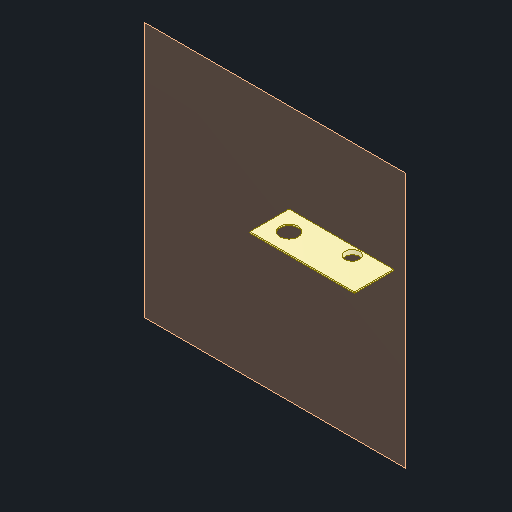
# Autodesk Inventor part: right_hold
Saved by Autodesk Inventor 2023 (Build 270158000, 158)
## iProperties
Created: 2024-05-18
Part Number: right_hold
Material: Nylon 6/6
Document SubType Name: Modeling
Designer: szymo
Density: 1.13 g/cm^3
Appearance: Nylon 6
Mass: 2.76791 g
Surface Area: 49.1971 cm^2
Volume: 2.44948 cm^3
Author: szymo
Autodesk Inventor part; units mm, degrees
ref_plane "YZ Plane" through (0, 0, 0) normal (1, 0, 0) x (0, 1, 0)
ref_plane "XZ Plane" through (0, 0, 0) normal (0, 1, 0) x (-1, 0, 0)
ref_plane "XY Plane" through (0, 0, 0) normal (0, 0, 1) x (1, 0, 0)
ref_plane "Work Plane1" through (0, 0, 0) normal (0, 0, 1) x (1, 0, 0)
sketch "Sketch1" plane through (0, 0, 0) normal (0, 0, 1) x (1, 0, 0)
  line L0 (-71, -74) -> (-71, -89) projected
  line L1 (-71, -89) -> (41, -89) projected
  line L2 (41, -89) -> (41, -30.5) projected
  line L3 (41, -30.5) -> (91, -30.5) projected
  line L4 (91, -30.5) -> (91, 30.5) projected
  line L5 (91, 30.5) -> (41, 30.5) projected
  line L6 (41, 30.5) -> (41, 89) projected
  line L7 (41, 89) -> (-71, 89) projected
  line L8 (-71, 89) -> (-71, 74) projected
  line L9 (-71, 74) -> (-87, 74) projected
  line L10 (-87, 74) -> (-87, 89) projected
  line L11 (-87, 89) -> (-91, 89) projected
  line L12 (-91, 89) -> (-91, -89) projected
  line L13 (-91, -89) -> (-87, -89) projected
  line L14 (-87, -89) -> (-87, -74) projected
  line L15 (-87, -74) -> (-71, -74) projected
  line L16 (91, 29.5) -> (11, 29.5)
  line L17 (11, 29.5) -> (11, 28.5)
  line L18 (11, 28.5) -> (91, 28.5)
  line L19 (91, 28.5) -> (91, 29.5)
  line L20 (71.5, 26) -> (60.5, 26) projected
  line L21 (12, 37) -> (40, 37) projected
  line L22 (11, 8.5) -> (11, 9.5)
  point P0 (0, 0)
  dimension "d0" = 1
  dimension "d1" = 2.5
  dimension "d2" = 1
  dimension "d14" = 0
  constraints: 10 end point, 2 parallel, 1 horizontal, 1 perpendicular, 1 point on line, 1 vertical, 2 other
  measures "d0" distance between parallel lines of L5 L16
  measures "d1" distance between parallel lines of L18 L20
  measures "d2" distance between parallel lines of L16 L18
  measures "d14" distance between parallel lines of L22 L17
ref_plane "Work Plane2" through (11, 8.5, 30) normal (0, 0, 1) x (1, 0, 0)
extrude "Extrusion1" add sketch "Sketch1" along normal up to surface (30 mm away) contours L18 L17 L16 L4
sketch "Sketch2" plane through (11, 28.5, 0) normal (0, -1, 0) x (1, 0, 0)
  circle A0 centre (55, 6.5) radius 5.5 projected
  arc A1 (12.5575, 17.9943) -> (10.6437, 18.8944) centre (9.6132, 14.2185) ccw projected
  arc A2 (10.6437, 18.8944) -> (10.0881, 18.165) centre (15, 15) ccw projected
  arc A3 (10.0881, 18.165) -> (11.4644, 16.5591) centre (14.322, 20.4008) ccw projected
  arc A4 (11.4644, 16.5591) -> (11.264, 15.9868) centre (15, 15) ccw projected
  arc A5 (11.264, 15.9868) -> (9.1866, 15.59) centre (11.1013, 11.2015) ccw projected
  arc A6 (9.1866, 15.59) -> (9.1659, 14.6734) centre (15, 15) ccw projected
  arc A7 (9.1659, 14.6734) -> (11.2232, 14.1831) centre (11.277, 18.9709) ccw projected
  arc A8 (11.2232, 14.1831) -> (11.3975, 13.6024) centre (15, 15) ccw projected
  arc A9 (11.3975, 13.6024) -> (9.95, 12.0603) centre (14.0786, 9.6353) ccw projected
  arc A10 (9.95, 12.0603) -> (10.4721, 11.3065) centre (15, 15) ccw projected
  arc A11 (10.4721, 11.3065) -> (12.4247, 12.1192) centre (9.654, 16.0242) ccw projected
  arc A12 (12.4247, 12.1192) -> (12.907, 11.7518) centre (15, 15) ccw projected
  arc A13 (12.907, 11.7518) -> (12.6424, 9.6535) centre (17.4078, 10.1183) ccw projected
  arc A14 (12.6424, 9.6535) -> (13.5078, 9.3505) centre (15, 15) ccw projected
  arc A15 (13.5078, 9.3505) -> (14.6098, 11.1556) centre (10.073, 12.6863) ccw projected
  arc A16 (14.6098, 11.1556) -> (15.216, 11.1419) centre (15, 15) ccw projected
  arc A17 (15.216, 11.1419) -> (16.2353, 9.2888) centre (19.8174, 12.4659) ccw projected
  arc A18 (16.2353, 9.2888) -> (17.1135, 9.5523) centre (15, 15) ccw projected
  arc A19 (17.1135, 9.5523) -> (16.944, 11.6605) centre (12.3739, 10.2321) ccw projected
  arc A20 (16.944, 11.6605) -> (17.4425, 12.0057) centre (15, 15) ccw projected
  arc A21 (17.4425, 12.0057) -> (19.3563, 11.1056) centre (20.3868, 15.7815) ccw projected
  arc A22 (19.3563, 11.1056) -> (19.9119, 11.835) centre (15, 15) ccw projected
  arc A23 (19.9119, 11.835) -> (18.5356, 13.4409) centre (15.678, 9.5992) ccw projected
  arc A24 (18.5356, 13.4409) -> (18.736, 14.0132) centre (15, 15) ccw projected
  arc A25 (18.736, 14.0132) -> (20.8134, 14.41) centre (18.8987, 18.7985) ccw projected
  arc A26 (20.8134, 14.41) -> (20.8341, 15.3266) centre (15, 15) ccw projected
  arc A27 (20.8341, 15.3266) -> (18.7768, 15.8169) centre (18.723, 11.0291) ccw projected
  arc A28 (18.7768, 15.8169) -> (18.6025, 16.3976) centre (15, 15) ccw projected
  arc A29 (18.6025, 16.3976) -> (20.05, 17.9397) centre (15.9214, 20.3647) ccw projected
  arc A30 (20.05, 17.9397) -> (19.5279, 18.6935) centre (15, 15) ccw projected
  arc A31 (19.5279, 18.6935) -> (17.5753, 17.8808) centre (20.346, 13.9758) ccw projected
  arc A32 (17.5753, 17.8808) -> (17.093, 18.2482) centre (15, 15) ccw projected
  arc A33 (17.093, 18.2482) -> (17.3576, 20.3465) centre (12.5922, 19.8817) ccw projected
  arc A34 (17.3576, 20.3465) -> (16.4922, 20.6495) centre (15, 15) ccw projected
  arc A35 (16.4922, 20.6495) -> (15.3902, 18.8444) centre (19.927, 17.3137) ccw projected
  arc A36 (15.3902, 18.8444) -> (14.784, 18.8581) centre (15, 15) ccw projected
  arc A37 (14.784, 18.8581) -> (13.7647, 20.7112) centre (10.1826, 17.5341) ccw projected
  arc A38 (13.7647, 20.7112) -> (12.8865, 20.4477) centre (15, 15) ccw projected
  arc A39 (12.8865, 20.4477) -> (13.056, 18.3395) centre (17.6261, 19.7679) ccw projected
  arc A40 (13.056, 18.3395) -> (12.5575, 17.9943) centre (15, 15) ccw projected
  circle A41 centre (15, 15) radius 5.8433
  circle A42 centre (15, 15) radius 7
  point P0 (-11, 0)
  dimension "d12" = 11.6865
  dimension "d13" = 14
  constraints: 2 centre point, 2 coincident
  measures "d12" diameter of A41
  measures "d13" diameter of A42
extrude "Extrusion2" cut sketch "Sketch2" against normal up to next contours A0 | A40 A39 A38 A37 A36 A35 A34 A33 A32 A31 A30 A29 A28 A27 A26 A25 A24 A23 A22 A21 A20 A19 A18 A17 A16 A15 A14 A13 A12 A11 A10 A9 A8 A7 A6 A5 A4 A3 A2 A1 | A1 A41 A39 A40 | A3 A4 A5 A41 | A41 A35 A36 A37 | A7 A8 A9 A41 | A41 A31 A32 A33 | A11 A12 A13 A41 | A41 A27 A28 A29 | A15 A16 A17 A41 | A19 A20 A21 A41 | A41 A23 A24 A25 | A42
sketch "Sketch3" plane through (11, 28.5, 0) normal (0, -1, 0) x (1, 0, 0)
  circle A0 centre (25.2408, 2.7067) radius 2 projected
  circle A1 centre (55, 6.5) radius 5.5 projected
  circle A2 centre (55, 6.5) radius 7.5
  circle A3 centre (25.2408, 2.7067) radius 4
  point P0 (-11, 0)
  dimension "d8" = 2
  dimension "d9" = 2
  constraints: 2 centre point
  measures "d8" radial gap between concentric circles of A1 A2
  measures "d9" radial gap between concentric circles of A0 A3
ref_plane "Work Plane3" through (58.3168, 26, -1.1832) normal (0, -1, 0) x (0.8086551, 0, -0.588283)
extrude "Extrusion3" add sketch "Sketch3" along normal up to surface (2.5 mm away)
body "Solid1"
